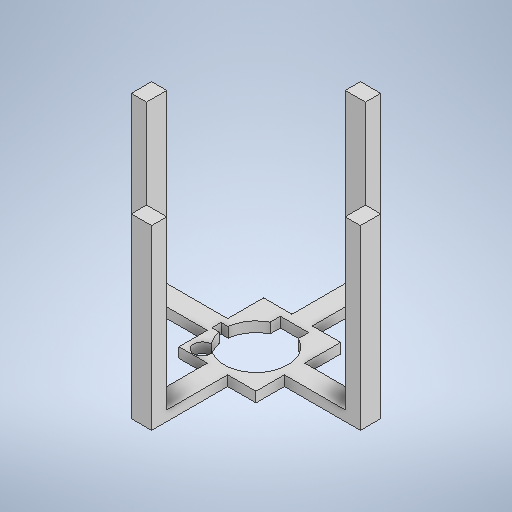
# Autodesk Inventor part: Camera Stand 2.0
Saved by Autodesk Inventor 2025 (Build 290162000, 162)
## iProperties
Created: 2024-06-13
Part Number: Camera Stand 2.0
Material: Generic
Document SubType Name: Modeling
Designer: agonzalez
Density: 1 g/cm^3
Appearance: Default
Author: agonzalez
Autodesk Inventor part; units mm, degrees
ref_plane "YZ Plane" through (0, 0, 0) normal (1, 0, 0) x (0, 1, 0)
ref_plane "XZ Plane" through (0, 0, 0) normal (0, 1, 0) x (-1, 0, 0)
ref_plane "XY Plane" through (0, 0, 0) normal (0, 0, 1) x (1, 0, 0)
sketch "Sketch1" plane through (0, 0, 0) normal (0, 1, 0) x (-1, 0, 0)
  line L0 (0, 0) -> (38.608, 0)
  line L1 (38.608, 0) -> (38.608, -38.608)
  line L2 (38.608, -38.608) -> (0, -38.608)
  line L3 (0, -38.608) -> (0, 0)
  dimension "d0" = 38.608
  dimension "d1" = 38.608
  constraints: 8 end point, 2 parallel, 1 horizontal, 1 perpendicular
  measures "d0" distance of L1.end L2.end
  measures "d1" distance of L0.end L1.end
extrude "Extrusion1" add sketch "Sketch1" along normal blind 5.08
sketch "Sketch2" plane through (0, 0, 0) normal (0, -1, 0) x (1, 0, 0)
  line L0 (-38.608, 0) -> (0, 0) projected
  circle A0 centre (-19.304, -19.304) radius 15.875
  line L1 (-38.608, -38.608) -> (-38.608, 0) projected
  line L2 (-38.608, -19.304) -> (-38.608, -21.082)
  line L3 (-38.608, -21.082) -> (-34.9151, -21.082)
  line L4 (-34.9151, -21.082) -> (-34.9151, -16.4216)
  line L5 (-34.9151, -16.4216) -> (-38.608, -16.4216)
  line L6 (-38.608, -16.4216) -> (-38.608, -21.082)
  line L7 (-19.304, -19.304) -> (-19.304, -38.608)
  line L8 (0, -38.608) -> (-38.608, -38.608) projected
  line L9 (-12.192, -31.75) -> (-12.192, -38.608)
  line L10 (-12.192, -38.608) -> (-26.416, -38.608)
  line L11 (-26.416, -38.608) -> (-26.416, -31.75)
  line L12 (-26.416, -31.75) -> (-12.192, -31.75)
  line L13 (-12.192, -31.75) -> (-26.416, -38.608) construction
  line L14 (-12.192, -38.608) -> (-26.416, -31.75) construction
  line L15 (-19.304, -19.304) -> (-0.2032, -19.304) construction
  circle A1 centre (-31.8453, -4.8972) radius 4.318
  point P0 (-35.0791, -21.082)
  point P1 (-19.304, -35.179)
  point P2 (-26.416, -33.4968)
  point P3 (-12.192, -33.4968)
  point P4 (-31.5527, -9.2053)
  point P5 (-27.6186, -5.7806)
  dimension "d4" = 31.75
  dimension "d8" = 14.224
  dimension "d11" = 8.636
  dimension "d42" = 6.858
  dimension "d43" = 3.6929
  dimension "d44" = 4.6604
  dimension "d45" = 3.6929
  constraints: 26 end point, 4 midpoint, 4 parallel, 3 perpendicular, 2 centre point, 2 horizontal, 2 point on circle, 2 point on line
  measures "d4" diameter of A0
  measures "d8" distance of L9.end L10.end
  measures "d11" diameter of A1
  measures "d42" distance of L10.end L11.end
  measures "d43" distance of L2.end L3.end
  measures "d44" distance of L3.end L4.end
  measures "d45" distance of L4.end L5.end
extrude "Extrusion2" cut sketch "Sketch2" against normal blind 6.35 contours A0 L9 L12 L11 L3 L4 A1 | A1 A0 | A0 A1 | L9 L8 L7 A0 | A0 L7 L12 L9 | L7 L8 L11 A0 | A0 L11 L12 L7 | L4 L3 A0 | A0 L3 L1 L5
sketch "Sketch4" plane through (0, 0, 0) normal (1, 0, 0) x (0, 0, -1)
  line L0 (38.608, 0) -> (38.608, 5.08) projected
  line L1 (0, 5.08) -> (38.608, 5.08) projected
  line L2 (12.954, 6.35) -> (25.654, 6.35)
  line L3 (14.224, 0) -> (14.224, 6.35)
  line L4 (14.224, 6.35) -> (24.384, 6.35)
  line L5 (24.384, 6.35) -> (24.384, 0)
  line L6 (24.384, 0) -> (14.224, 0)
  line L7 (14.224, 0) -> (24.384, 6.35) construction
  line L8 (14.224, 6.35) -> (24.384, 0) construction
  point P0 (0, 0)
  point P1 (19.304, 3.175)
  point P2 (24.384, 5.08)
  point P3 (14.224, 5.08)
  dimension "d19" = 10.16
  constraints: 14 end point, 2 midpoint, 2 parallel, 1 perpendicular
  measures "d19" distance of L3.end L4.end
extrude "Extrusion4" add sketch "Sketch4" along normal blind 38.1 contours L1 L5 L6 L3
sketch "Sketch6" plane through (-38.608, 0, 0) normal (0, 0, 1) x (1, 0, 0)
  line L0 (0, 0) -> (3.6929, 0) projected
  line L1 (38.608, 5.08) -> (76.708, 5.08) projected
  line L2 (0, 0) -> (0, 5.08) projected
  line L3 (38.608, 0) -> (76.708, 0) projected
  line L4 (0, 5.08) -> (38.608, 5.08) projected
  line L5 (24.384, 5.08) -> (14.224, 5.08)
  line L6 (0, 0) -> (38.608, 0) projected
  line L7 (14.224, 0) -> (24.384, 0)
  line L8 (24.384, 0) -> (24.384, 5.08)
  line L9 (24.384, 5.08) -> (14.224, 5.08)
  line L10 (14.224, 5.08) -> (14.224, 0)
  line L11 (14.224, 0) -> (24.384, 5.08) construction
  line L12 (24.384, 0) -> (14.224, 5.08) construction
  point P0 (19.304, 2.54)
  dimension "d24" = 10.16
  constraints: 14 end point, 2 midpoint, 2 parallel, 1 horizontal, 1 perpendicular, 1 point on line
  measures "d24" distance of L9.end L5.start
sketch "Sketch7" plane through (-38.608, 0, -38.608) normal (-1, 0, 0) x (0, 0, 1)
  line L0 (0, 0) -> (0, 5.08) projected
  line L1 (22.1864, 0) -> (38.608, 0) projected
  line L2 (22.1864, 5.08) -> (38.608, 5.08) projected
  line L3 (38.608, 0) -> (38.608, 5.08) projected
  line L4 (5.1112, 5.08) -> (35.179, 5.08) projected
  line L5 (24.384, 0) -> (14.224, 0)
  line L6 (14.224, 0) -> (14.224, 5.08)
  line L7 (14.224, 5.08) -> (24.384, 5.08)
  line L8 (24.384, 5.08) -> (24.384, 0)
  line L9 (24.384, 0) -> (14.224, 5.08) construction
  line L10 (14.224, 0) -> (24.384, 5.08) construction
  point P0 (32.8274, 5.08)
  point P1 (19.304, 2.54)
  dimension "d25" = 10.16
  constraints: 12 end point, 2 midpoint, 2 parallel, 1 horizontal, 1 perpendicular, 1 point on line
  measures "d25" distance of L6.end L7.end
extrude "Extrusion5" add sketch "Sketch6" along normal blind 38.1 contours L10 L4 L8 L6
extrude "Extrusion6" add sketch "Sketch7" along normal blind 38.1 contours L5 L6 L4 L2 L8 L1
sketch "Sketch8" plane through (0, 0, -38.608) normal (0, 0, -1) x (-1, 0, 0)
  line L0 (0, 0) -> (0, 5.08) projected
  line L1 (38.608, 0) -> (34.9151, 0) projected
  line L2 (0, 5.08) -> (38.608, 5.08)
  line L3 (38.608, 5.08) -> (38.608, 0)
  line L4 (38.608, 0) -> (0, 0)
  line L5 (0, 0) -> (0, 5.08)
  constraints: 8 end point, 2 parallel, 1 horizontal, 1 perpendicular
extrude "Extrusion7" add sketch "Sketch8" along normal blind 3.81
sketch "Sketch9" plane through (0, 0, -42.418) normal (0, 0, -1) x (-1, 0, 0)
  line L0 (38.608, 5.08) -> (0, 5.08) projected
  line L1 (38.608, 0) -> (76.708, 0) projected
  line L2 (3.429, 5.08) -> (27.6186, 5.08) projected
  line L3 (14.224, 0) -> (24.384, 0)
  line L4 (24.384, 0) -> (24.384, 5.08)
  line L5 (24.384, 5.08) -> (14.224, 5.08)
  line L6 (14.224, 5.08) -> (14.224, 0)
  line L7 (14.224, 0) -> (24.384, 5.08) construction
  line L8 (24.384, 0) -> (14.224, 5.08) construction
  point P0 (0, 0)
  point P1 (12.192, 5.08)
  point P2 (19.304, 2.54)
  point P3 (14.224, 5.08)
  dimension "d32" = 10.16
  constraints: 12 end point, 2 midpoint, 2 parallel, 1 horizontal, 1 perpendicular, 1 point on line
  measures "d32" distance of L5.end L4.end
extrude "Extrusion8" add sketch "Sketch9" along normal blind 34.29
sketch "Sketch10" plane through (0, 5.08, 0) normal (0, 1, 0) x (1, 0, 0)
  line L0 (-76.708, 24.384) -> (-76.708, 14.224) projected
  line L1 (-38.608, 24.384) -> (-76.708, 24.384) projected
  line L2 (-76.708, 14.224) -> (-69.088, 14.224)
  line L3 (-69.088, 14.224) -> (-69.088, 24.384)
  line L4 (-69.088, 24.384) -> (-76.708, 24.384)
  line L5 (-76.708, 24.384) -> (-76.708, 14.224)
  line L6 (-14.224, 76.708) -> (-24.384, 76.708) projected
  line L7 (-14.224, 76.708) -> (-24.384, 76.708)
  line L8 (-24.384, 76.708) -> (-24.384, 69.088)
  line L9 (-24.384, 69.088) -> (-14.224, 69.088)
  line L10 (-14.224, 69.088) -> (-14.224, 76.708)
  line L11 (38.1, 14.224) -> (38.1, 24.384) projected
  line L12 (0, 24.384) -> (38.1, 24.384) projected
  line L13 (38.1, 14.224) -> (30.48, 14.224)
  line L14 (30.48, 14.224) -> (30.48, 24.384)
  line L15 (30.48, 24.384) -> (38.1, 24.384)
  line L16 (38.1, 24.384) -> (38.1, 14.224)
  line L17 (-14.224, 0) -> (-14.224, -38.1) projected
  line L18 (-24.384, 0) -> (-24.384, -38.1) projected
  line L19 (-14.224, -38.1) -> (-24.384, -38.1)
  line L20 (-24.384, -38.1) -> (-24.384, -30.48)
  line L21 (-24.384, -30.48) -> (-14.224, -30.48)
  line L22 (-14.224, -30.48) -> (-14.224, -38.1)
  point P0 (0, 0)
  dimension "d35" = 7.62
  dimension "d36" = 10.16
  dimension "d37" = 7.62
  dimension "d38" = 7.62
  dimension "d39" = 7.62
  constraints: 32 end point, 8 parallel, 4 horizontal, 4 perpendicular, 3 point on line
  measures "d35" distance of L4.end L3.end
  measures "d36" distance of L9.end L8.end
  measures "d37" distance of L8.end L7.end
  measures "d38" distance of L14.end L15.end
  measures "d39" distance of L19.end L20.end
extrude "Extrusion9" add sketch "Sketch10" along normal blind 83.82
body "Solid1"
